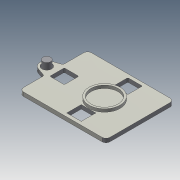
# Autodesk Inventor part: cover
Saved by Autodesk Inventor 2015 (Build 190159000, 159)
## iProperties
Created: 2017-05-03
Part Number: cover
Material: 일반
Document SubType Name: Modeling
Designer: gatew
Density: 1 g/cm^3
Appearance: 기본값
Author: gatew
Autodesk Inventor part; units mm, degrees
ref_plane "YZ Plane" through (0, 0, 0) normal (1, 0, 0) x (0, 1, 0)
ref_plane "XZ Plane" through (0, 0, 0) normal (0, 1, 0) x (-1, 0, 0)
ref_plane "XY Plane" through (0, 0, 0) normal (0, 0, 1) x (1, 0, 0)
sketch "스케치1" plane through (0, 0, 0) normal (0, 1, 0) x (-1, 0, 0)
  line L0 (35, 52.5) -> (-35, 52.5)
  line L1 (-35, 52.5) -> (-35, -52.5)
  line L2 (-35, -52.5) -> (35, -52.5)
  line L3 (35, -52.5) -> (35, 52.5)
  line L4 (35, 52.5) -> (-35, -52.5) construction
  line L5 (-35, 52.5) -> (35, -52.5) construction
  point P0 (0, 0)
  dimension "d0" = 70
  dimension "d1" = 105
  constraints: 12 end point, 2 midpoint, 2 parallel, 1 horizontal, 1 perpendicular
  measures "d0" distance of L2.end L1.end
  measures "d1" distance of L1.end L0.end
extrude "돌출1" add sketch "스케치1" along normal blind 4
fillet "모깎기1" radius 4 4 edges at (-35, 2, 52.5) (35, 2, 52.5) (35, 2, -52.5) (-35, 2, -52.5)
sketch "스케치12" plane through (0, 4, 0) normal (0, 1, 0) x (1, 0, 0)
  circle A0 centre (0, 0) radius 14
  circle A1 centre (0, 0) radius 16
  dimension "d80" = 28
  dimension "d81" = 2
  constraints: 2 centre point, 1 coincident
  measures "d80" diameter of A0
  measures "d81" radial gap between concentric circles of A0 A1
extrude "돌출9" add sketch "스케치12" along normal blind 3
sketch "스케치13" plane through (0, 4, 0) normal (0, 1, 0) x (1, 0, 0)
  arc A0 (-6.6134, -61.794) -> (6.6134, -61.794) centre (0, -59.5) ccw
  line L0 (-31, -52.5) -> (31, -52.5) projected
  circle A1 centre (0, -59.5) radius 5
  line L1 (-6.6134, -61.794) -> (-9.8372, -52.5)
  line L2 (-31, -52.5) -> (31, -52.5) projected
  line L3 (6.6134, -61.794) -> (9.8372, -52.5)
  line L4 (-9.8372, -52.5) -> (9.8372, -52.5)
  point P0 (0, 0)
  dimension "d84" = 14
  dimension "d85" = 7
  dimension "d86" = 10
  dimension "d87" = 0
  constraints: 6 end point, 2 centre point, 2 point on circle, 1 coincident, 1 collinear, 1 point on line, 1 tangent
  measures "d84" diameter of A0
  measures "d85" distance from line of L0 A0.centre
  measures "d86" diameter of A1
  measures "d87" horizontal distance of point (0, 0) A0.centre
extrude "돌출10" add sketch "스케치13" against normal up to surface (4 mm away) contours L1 L0 L3 A0 | A1
sketch "스케치14" plane through (0, 4, 0) normal (0, 1, 0) x (1, 0, 0)
  circle A0 centre (0, -59.5) radius 5
  line L0 (9.8372, -52.5) -> (31, -52.5) projected
  point P0 (0, 0)
  dimension "d90" = 10
  dimension "d91" = 7
  constraints: 1 centre point
  measures "d90" diameter of A0
  measures "d91" distance from line of L0 A0.centre
extrude "돌출11" cut sketch "스케치14" against normal blind 3
sketch "스케치15" plane through (0, 1, 59.5) normal (0, 1, 0) x (1, 0, 0)
  circle A0 centre (0, 0) radius 4
  point P0 (0, 59.5)
  dimension "d94" = 8
  constraints: 1 centre point
  measures "d94" diameter of A0
extrude "돌출12" add sketch "스케치15" along normal blind 9
fillet "모깎기14" radius 2 2 edges at (9.8372, 2, 52.5) (-9.8372, 2, 52.5)
mirror "대칭2" about plane through (0, 0, 0) normal (0, 0, 1) of "돌출10", "돌출12", "돌출11"
fillet "모깎기15" radius 2 2 edges at (9.8372, 2, -52.5) (-9.8372, 2, -52.5)
sketch "스케치16" plane through (0, 4, 0) normal (0, 1, 0) x (1, 0, 0)
  line L0 (-31, -52.5) -> (-11.2604, -52.5) projected
  line L1 (31, 52.5) -> (11.2604, 52.5) projected
  line L2 (-35, 48.5) -> (-35, -48.5) projected
  line L3 (-7.5, -49) -> (7.5, -49)
  line L4 (7.5, -49) -> (7.5, -34)
  line L5 (7.5, -34) -> (-7.5, -34)
  line L6 (-7.5, -34) -> (-7.5, -49)
  line L7 (-7.5, -49) -> (7.5, -34) construction
  line L8 (7.5, -49) -> (-7.5, -34) construction
  line L9 (11.2604, -52.5) -> (31, -52.5) projected
  line L10 (-31.5, -7.5) -> (-16.5, -7.5)
  line L11 (-16.5, -7.5) -> (-16.5, 7.5)
  line L12 (-16.5, 7.5) -> (-31.5, 7.5)
  line L13 (-31.5, 7.5) -> (-31.5, -7.5)
  line L14 (-31.5, -7.5) -> (-16.5, 7.5) construction
  line L15 (-16.5, -7.5) -> (-31.5, 7.5) construction
  line L16 (31.5, -7.5) -> (16.5, -7.5)
  line L17 (16.5, -7.5) -> (16.5, 7.5)
  line L18 (16.5, 7.5) -> (31.5, 7.5)
  line L19 (31.5, 7.5) -> (31.5, -7.5)
  point P0 (0, 0)
  point P1 (0, -41.5)
  point P2 (-24, 0)
  point P3 (24, 0)
  dimension "d110" = 15
  dimension "d111" = 15
  dimension "d112" = 11
  dimension "d113" = 15
  dimension "d114" = 15
  dimension "d115" = 11
  constraints: 32 end point, 4 midpoint, 4 parallel, 2 horizontal, 2 perpendicular
  measures "d110" distance of L5.end L4.end
  measures "d111" distance of L4.end L3.end
  measures "d112" distance from line of L9 point (0, -41.5)
  measures "d113" distance of L12.end L11.end
  measures "d114" distance of L11.end L10.end
  measures "d115" distance from line of L2 point (-24, 0)
extrude "돌출13" cut sketch "스케치16" against normal blind 10
fillet "모깎기16" radius 1 7 edges at (-7.5, 2, 49) (-7.5, 2, 34) (7.5, 2, 34) (7.5, 2, 49) (-16.5, 2, 7.5) (-31.5, 2, 7.5) (-16.5, 2, -7.5)
fillet "모깎기17" radius 1 1 edges at (-31.5, 2, -7.5)
sketch "스케치17" plane through (-31, 0, -52.5) normal (0, 0, -1) x (-1, 0, 0)
  line L0 (-73.5651, 25.0747) -> (54.285, 25.0747)
  line L1 (54.285, 25.0747) -> (54.285, -23.2173)
  line L2 (54.285, -23.2173) -> (-73.5651, -23.2173)
  line L3 (-73.5651, -23.2173) -> (-73.5651, 25.0747)
  line L4 (-73.5651, 25.0747) -> (54.285, -23.2173) construction
  line L5 (54.285, 25.0747) -> (-73.5651, -23.2173) construction
  point P0 (-31, 0)
  point P1 (-9.6401, 0.9287)
  constraints: 12 end point, 2 midpoint, 2 parallel, 1 horizontal, 1 perpendicular
extrude "돌출14" cut sketch "스케치17" against normal blind 20
extrude "돌출15" cut sketch "스케치17" along normal blind 20
sketch "스케치18" plane through (0, 4, 0) normal (0, 1, 0) x (1, 0, 0)
  line L0 (-35, 32.5) -> (35, 32.5)
  line L1 (-35, 32.5) -> (-35, 32.5)
  line L2 (-31, 36.5) -> (31, 36.5)
  line L3 (35, 32.5) -> (35, 32.5)
  arc A0 (35, 32.5) -> (31, 36.5) centre (31, 32.5) ccw
  arc A1 (-31, 36.5) -> (-35, 32.5) centre (-31, 32.5) ccw
  point P0 (0, 0)
  point P1 (-35, 36.5)
  dimension "d125" = 70
  dimension "d126" = 4
  dimension "d127" = 4
  constraints: 8 end point, 4 point on circle, 4 tangent, 2 centre point, 2 perpendicular, 2 point on line, 1 equal radius, 1 horizontal, 1 vertical
  measures "d125" distance of L0.start L0.end
  measures "d126" distance of L0.start point (-35, 36.5)
  measures "d127" radius of A0
extrude "돌출16" add sketch "스케치18" against normal up to surface (4 mm away)
